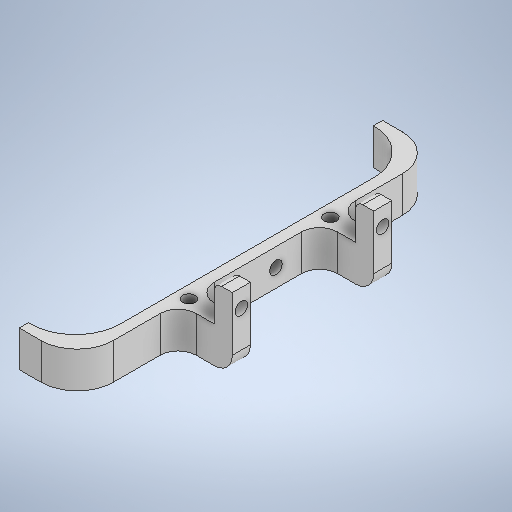
# Autodesk Inventor part: pare-chocs
Saved by Autodesk Inventor 2025 (Build 290162000, 162)
## iProperties
Created: 2024-09-30
Part Number: pare-chocs
Material: Générique
Document SubType Name: Modeling
Designer: chass
Density: 1 g/cm^3
Appearance: Par défaut
Author: chass
Autodesk Inventor part; units mm, degrees
ref_plane "YZ Plane" through (0, 0, 0) normal (1, 0, 0) x (0, 1, 0)
ref_plane "XZ Plane" through (0, 0, 0) normal (0, 1, 0) x (-1, 0, 0)
ref_plane "XY Plane" through (0, 0, 0) normal (0, 0, 1) x (1, 0, 0)
sketch "Esquisse1" plane through (0, 0, 0) normal (0, 1, 0) x (-1, 0, 0)
  line L0 (-1.5, 50) -> (1.5, 50)
  line L1 (1.5, 50) -> (1.5, -50)
  line L2 (1.5, -50) -> (-1.5, -50)
  line L3 (-1.5, -50) -> (-1.5, 50)
  line L4 (1.5, 50) -> (-1.5, -50)
  line L5 (-1.5, 50) -> (1.5, -50)
  circle A0 centre (14, -35) radius 12.5
  line L6 (-10, 0) -> (16, 0)
  circle A1 centre (14, 35) radius 12.5
  line L7 (1.5, -50) -> (14, -50)
  line L8 (14, -50) -> (14, -47.5)
  line L9 (9, -23.5436) -> (9, 23.5436)
  line L10 (1.5, 50) -> (14.5259, 50)
  line L11 (14.5259, 50) -> (14.5259, 47.4889)
  point P0 (0, 0)
  point P1 (0, 0)
  point P2 (0, 0)
  point P3 (14, -22.5)
  point P4 (14, 22.5)
  point P5 (1.5, 35)
  point P6 (1.5, -35)
  dimension "d0" = 3
  dimension "d1" = 100
  dimension "d19" = 25
  constraints: 24 end point, 6 point on circle, 4 horizontal, 3 parallel, 2 centre point, 2 midpoint, 2 perpendicular, 1 coincident, 1 symmetric about line, 1 vertical, 1 other
  measures "d0" distance of L1.end L2.end
  measures "d1" distance of L0.end L1.end
  measures "d19" diameter of A0
extrude "Extrusion1" add sketch "Esquisse1" along normal blind 10 contours L5 L6 L3 | L0 L4 L5 | L10 L11 A1 L1 | L1 L6 L4 | L6 L4 L3 | L5 L2 L4 | L6 L1 L5 | L1 A0 L8 L7
sketch "Esquisse2" plane through (1.5, 0, 50) normal (1, 0, 0) x (0, 0, -1)
  line L0 (0, 0) -> (100, 0) projected
  line L1 (27.9472, 0) -> (32.9472, 0)
  line L2 (32.9472, 0) -> (32.9472, 10)
  line L3 (32.9472, 10) -> (27.9472, 10)
  line L4 (27.9472, 10) -> (27.9472, 0)
  line L5 (50, 0) -> (50, 10.1076)
  line L6 (67.0528, 0) -> (67.0528, 10)
  line L7 (67.0528, 10) -> (72.0528, 10)
  line L8 (72.0528, 10) -> (72.0528, 0)
  dimension "d4" = 5
  dimension "d5" = 10
  constraints: 16 end point, 4 symmetric about line, 2 parallel, 1 horizontal, 1 perpendicular, 1 point on line, 1 vertical
  measures "d4" distance of L3.end L2.end
  measures "d5" distance of L2.end L1.end
extrude "Extrusion2" add sketch "Esquisse2" along normal blind 15
fillet "Congé1" radius 10 2 edges at (1.5, 5, -50) (1.5, 5, 50)
sketch "Esquisse5" plane through (0, 10, 0) normal (0, 1, 0) x (1, 0, 0)
  line L0 (16.5, 17.0528) -> (16.5, 22.0528) projected
  line L1 (1.5, 17.0528) -> (16.5, 17.0528) projected
  line L2 (16.5, 22.0528) -> (11.5, 22.0528)
  line L3 (11.5, 22.0528) -> (11.5, 17.0528)
  line L4 (11.5, 17.0528) -> (16.5, 17.0528)
  line L5 (16.5, 17.0528) -> (16.5, 22.0528)
  line L6 (-9, 0) -> (10, 0)
  line L7 (16.5, -17.0528) -> (16.5, -22.0528)
  line L8 (16.5, -22.0528) -> (11.5, -22.0528)
  line L9 (11.5, -22.0528) -> (11.5, -17.0528)
  line L10 (11.5, -17.0528) -> (16.5, -17.0528)
  line L11 (16.5, -17.0528) -> (16.5, -22.0528)
  point P0 (0, 0)
  dimension "d22" = 5
  constraints: 20 end point, 5 symmetric about line, 2 horizontal, 2 parallel, 1 perpendicular, 1 point on line
  measures "d22" distance of L4.end L3.end
extrude "Extrusion5" add sketch "Esquisse5" along normal blind 10
sketch "Esquisse6" plane through (16.5, 0, 50) normal (1, 0, 0) x (0, 0, -1)
  circle A0 centre (30.4472, 15) radius 1.75
  line L0 (27.9472, 20) -> (32.9472, 20) projected
  line L1 (27.9472, 0) -> (27.9472, 20) projected
  line L2 (50, 0) -> (50, 10)
  circle A1 centre (69.5528, 15) radius 1.75
  point P0 (30.4472, 20)
  dimension "d25" = 3.5
  dimension "d26" = 5
  dimension "d27" = 2.5
  constraints: 2 centre point, 2 end point, 1 midpoint, 1 symmetric about line, 1 vertical, 1 other
  measures "d25" diameter of A0
  measures "d26" distance of point (30.447, 20) A0.centre
  measures "d27" distance from line of L1 A0.centre
extrude "Extrusion6" cut sketch "Esquisse6" against normal blind 10
fillet "Congé2" radius 5 6 edges at (16.5, 0, 19.5528) (16.5, 0, -19.5528) (1.5, 5, 22.0528) (1.5, 5, -22.0528) (1.5, 5, -17.0528) (1.5, 5, 17.0528)
fillet "Congé3" radius 2 2 edges at (11.5, 20, 19.5528) (11.5, 20, -19.5528)
sketch "Esquisse7" plane through (0, 10, 0) normal (0, 1, 0) x (1, 0, 0)
  circle A0 centre (2, 19.5528) radius 1.75
  line L0 (-3.6278, 0) -> (5, 0)
  circle A1 centre (2, -19.5528) radius 1.75
  line L1 (6.5, 22.0528) -> (11.5, 22.0528) projected
  point P0 (0, 0)
  dimension "d32" = 3.5
  dimension "d33" = 2.5
  constraints: 2 centre point, 2 end point, 1 horizontal, 1 symmetric about line, 1 other
  measures "d32" diameter of A0
  measures "d33" distance from line of L1 A0.centre
extrude "Extrusion7" cut sketch "Esquisse7" against normal blind 23
sketch "Esquisse8" plane through (1.5, 0, 12.0528) normal (1, 0, 0) x (0, 0, -1)
  circle A0 centre (7.0528, 5) radius 1.75
  line L0 (12.0528, 0) -> (12.0528, 10)
  circle A1 centre (17.0528, 5) radius 1.75
  point P0 (12.0528, 5)
  dimension "d36" = 3.5
  dimension "d37" = 5
  constraints: 2 centre point, 2 end point, 1 midpoint, 1 symmetric about line, 1 vertical, 1 other
  measures "d36" diameter of A0
  measures "d37" distance of point (12.053, 5) A0.centre
extrude "Extrusion8" cut sketch "Esquisse8" against normal blind 3
